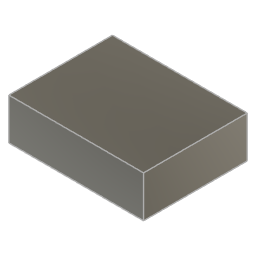
mounting brick (Autodesk Fusion 360 design; units mm, degrees)
Autodesk Fusion 360 part; units mm, degrees
sketch "Sketch1" plane through (0, 0, 0) normal (0, 0, 1) x (1, 0, 0)
  line L0 (0, 0) -> (70, 0)
  line L1 (70, 0) -> (70, 54.9797)
  line L2 (70, 54.9797) -> (0, 54.9797)
  line L3 (0, 54.9797) -> (0, 0)
  dimension "d1" = 70
  constraint horizontal L0
  constraint vertical L1
  constraint horizontal L2
  constraint vertical L3
  constraint coincident L0.start L3.end
  measures "d1" distance of L0.start L0.end
extrude "Extrude1" add sketch "Sketch1" along normal blind 20
move_face "OffsetFaces1" offset -5 2 faces at (70, 18.3266, 6.6667) (23.3333, 0, 6.6667)
